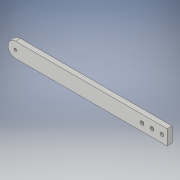
# Autodesk Inventor part: Wheel Arms
Saved by Autodesk Inventor 2019 (Build 230136000, 136)
## iProperties
Created: 2019-10-05
Part Number: Wheel Arms
Material: Generic
Document SubType Name: Modeling
Designer: Delta
Density: 1 g/cm^3
Appearance: Default
Author: Delta
Autodesk Inventor part; units mm, degrees
ref_plane "YZ Plane" through (0, 0, 0) normal (1, 0, 0) x (0, 1, 0)
ref_plane "XZ Plane" through (0, 0, 0) normal (0, 1, 0) x (-1, 0, 0)
ref_plane "XY Plane" through (0, 0, 0) normal (0, 0, 1) x (1, 0, 0)
sketch "Sketch1" plane through (0, 0, 0) normal (0, 0, 1) x (1, 0, 0)
  line L0 (0, 0) -> (203.2, 0)
  line L1 (203.2, 0) -> (203.2, -19.05)
  line L2 (203.2, -19.05) -> (0, -19.05)
  line L3 (0, -19.05) -> (0, 0)
  dimension "d0" = 203.2
  dimension "d1" = 19.05
  constraints: 8 end point, 2 parallel, 1 horizontal, 1 perpendicular
  measures "d0" distance of L1.end L2.end
  measures "d1" distance of L0.end L1.end
extrude "Extrusion1" add sketch "Sketch1" along normal blind 6.35
fillet "Fillet1" radius 9.525 2 edges at (0, -19.05, 3.175) (0, 0, 3.175)
sketch "Sketch4" plane through (0, 0, 6.35) normal (0, 0, 1) x (1, 0, 0)
  arc A0 (9.525, 0) -> (9.525, -19.05) centre (9.525, -9.525) ccw projected
  circle A1 centre (9.525, -9.525) radius 1.778
  point P0 (0, 0)
  point P1 (254, 0)
  point P2 (254, -19.05)
  dimension "d14" = 3.556
  constraints: 1 centre point, 1 coincident, 1 other
  measures "d14" diameter of A1
extrude "Extrusion4" cut sketch "Sketch4" against normal blind 12.7
sketch "Sketch5" plane through (0, 0, 6.35) normal (0, 0, 1) x (1, 0, 0)
  line L0 (9.525, -19.05) -> (203.2, -19.05) projected
  line L1 (203.2, 0) -> (9.525, 0) projected
  line L2 (203.2, -19.05) -> (203.2, 0) projected
  circle A0 centre (171.45, -9.525) radius 2.3368
  circle A1 centre (184.15, -9.525) radius 2.3368
  circle A2 centre (196.85, -9.525) radius 2.3368
  point P0 (0, 0)
  dimension "d17" = 19.05
  dimension "d18" = 9.525
  dimension "d19" = 19.05
  dimension "d20" = 9.525
  dimension "d21" = 12.7
  dimension "d22" = 4.6736
  dimension "d23" = 4.6736
  dimension "d28" = 12.7
  dimension "d29" = 4.6736
  dimension "d30" = 9.525
  constraints: 3 centre point, 3 coincident
  measures "d17" distance between parallel lines of L0 L1
  measures "d18" distance from line of L1 point (184.15, -9.525)
  measures "d19" distance from line of L2 point (184.15, -9.525)
  measures "d20" distance from line of L1 point (171.45, -9.525)
  measures "d21" distance of point (184.15, -9.525) point (171.45, -9.525)
  measures "d22" diameter of A0
  measures "d23" diameter of A1
  measures "d28" distance of A1.centre point (196.85, -9.525)
  measures "d29" diameter of A2
  measures "d30" distance from line of L0 point (196.85, -9.525)
extrude "Extrusion5" cut sketch "Sketch5" against normal through all
equation "\"d18\" = 0.5 * d17"
equation "\"d20\" = d18"
equation "\"d22\" = d23"
equation "\"d28\" = d21"
equation "\"d29\" = d22"
body "Solid1"
